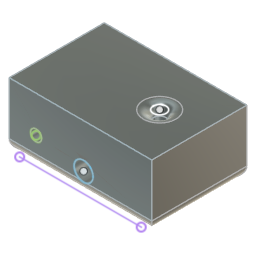
shuttle v5 (Autodesk Fusion 360 design; units mm, degrees)
Autodesk Fusion 360 part; units mm, degrees
sketch "Sketch1" plane through (0, 0, 0) normal (0, 0, 1) x (1, 0, 0)
  line L0 (0, 0) -> (114.3, 0)
  line L1 (114.3, 0) -> (114.3, -76.2)
  line L2 (114.3, -76.2) -> (0, -76.2)
  line L3 (0, -76.2) -> (0, 0)
  dimension "d1" = 114.3
  dimension "d2" = 76.2
  constraint horizontal L0
  constraint vertical L1
  constraint horizontal L2
  constraint vertical L3
  constraint coincident L0.start L3.end
  measures "d1" distance of L0.start L0.end
  measures "d2" distance of L0.start L2.end
extrude "Extrude1" add sketch "Sketch1" along normal blind 50.8
sketch "Sketch2" plane through (0, 0, 50.8) normal (0, 0, 1) x (-1, 0, 0)
  line L0 (0, 76.2) -> (-114.3, 76.2)
  line L1 (-114.3, 76.2) -> (-114.3, 0)
  line L2 (-114.3, 0) -> (0, 0)
  line L3 (0, 0) -> (0, 76.2)
  circle A0 centre (-82.55, 38.1) radius 5.08
  dimension "d5" = 10.16
  dimension "d6" = 38.1
  dimension "d7" = 31.75
  measures "d5" diameter of A0
  measures "d6" distance of L2 A0.centre
  measures "d7" distance of L1 A0.centre
extrude "Extrude2" cut sketch "Sketch2" against normal blind 50.8 contours A0
fillet "Fillet1" radius 7.9756 1 edges at (87.2862, -39.937, 50.8)
fillet "Fillet2" radius 8.4339 4 edges at (114.3, -38.1, 0) (57.15, -76.2, 0) (0, -38.1, 0) (57.15, 0, 0)
sketch "Sketch3" plane through (0, -76.2, 0) normal (0, -1, 0) x (1, 0, 0)
  line L0 (0, 8.4339) -> (114.3, 8.4339)
  line L1 (114.3, 8.4339) -> (114.3, 50.8)
  line L2 (114.3, 50.8) -> (0, 50.8)
  line L3 (0, 50.8) -> (0, 8.4339)
  circle A0 centre (21.59, 21.59) radius 4.445
  line L4 (8.4339, 0) -> (105.8661, 0)
  circle A1 centre (59.69, 15.6948) radius 7.62
  dimension "d20" = 8.89
  dimension "d21" = 21.59
  dimension "d22" = 21.59
  dimension "d23" = 15.24
  dimension "d24" = 59.69
  measures "d20" diameter of A0
  measures "d21" distance of L3 A0.centre
  measures "d22" distance of A0.centre L4
  measures "d23" diameter of A1
  measures "d24" distance of L3 A1.centre
extrude "Extrude4" cut sketch "Sketch3" against normal blind 76.2 contours L0 A1 | L0 A1
extrude "Extrude5" cut sketch "Sketch3" against normal blind 76.2 contours A0
